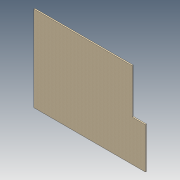
# Autodesk Inventor part: GE-12103-05
Saved by Autodesk Inventor 2012 (Build 160160000, 160)
## iProperties
Created: 2011-10-10
Part Number: GE-12103-05
Document SubType Name: Modeling
Designer: dfoster
Density: 1 g/cm^3
Description: Top, Plywood
Material: Default
Title: Top, Plywood
Author: dfoster
Autodesk Inventor part; units mm, degrees
ref_plane "YZ Plane" through (0, 0, 0) normal (1, 0, 0) x (0, 1, 0)
ref_plane "XZ Plane" through (0, 0, 0) normal (0, 1, 0) x (-1, 0, 0)
ref_plane "XY Plane" through (0, 0, 0) normal (0, 0, 1) x (1, 0, 0)
sketch "Sketch1" plane through (0, 0, 0) normal (0, 0, 1) x (1, 0, 0)
  line L0 (0, 0) -> (1276.35, 0)
  line L1 (1276.35, 0) -> (1276.35, 469.9)
  line L2 (1123.95, 977.9) -> (0, 977.9)
  line L3 (0, 977.9) -> (0, 0)
  line L4 (1123.95, 977.9) -> (1123.95, 469.9)
  line L5 (1123.95, 469.9) -> (1276.35, 469.9)
  dimension "d0" = 1276.35
  dimension "d1" = 977.9
  dimension "d2" = 1123.95
  dimension "d3" = 508
  constraints: 12 end point, 3 parallel, 2 perpendicular, 1 horizontal
  measures "d0" distance of L0.start L0.end
  measures "d1" distance of L2.end L0.start
  measures "d2" distance between parallel lines of L4 L3
  measures "d3" distance between parallel lines of L5 L2
extrude "Extrusion1" add sketch "Sketch1" along normal blind 12.7
body "Solid1"
